Autodesk Fusion 360 part; units mm, degrees
(part 4 of 7)
extrude "USB nose reference rectangular stock" add sketch "USB nose reference rectangular stock sketch" along normal blind 1.1 separate body makes body 51 in component "USB A3 — GCT USB4720 shell drawing reconstruction"
fillet "USB nose reference corner rounds" radius 1.05 4 edges at (38.33, 1.55, 24.72) (46.67, 1.55, 24.72) (46.67, 1.55, 27.28) (38.33, 1.55, 27.28) on bodies 51 in component "USB A3 — GCT USB4720 shell drawing reconstruction"
combine "USB nose reference" operation add target body 50 tool bodies 51 in component "USB A3 — GCT USB4720 shell drawing reconstruction"
ref_plane "WorkPlane3" through (0, 2.1, 0) normal (0, 1, 0) x (0, 0, 1) in component "USB A3 — GCT USB4720 shell drawing reconstruction"
sketch "USB shell rear cavity simplified rectangular stock sketch" plane through (0, 2.1, 0) normal (0, 1, 0) x (1, 0, 0) in component "USB A3 — GCT USB4720 shell drawing reconstruction"
  line L0 (38.53, -27.43) -> (46.47, -27.43)
  line L1 (46.47, -27.43) -> (46.47, -24.57)
  line L2 (46.47, -24.57) -> (38.53, -24.57)
  line L3 (38.53, -24.57) -> (38.53, -27.43)
  dimension "d1272" = 38.53
  dimension "d1273" = 27.43
  dimension "d1274" = 7.94
  dimension "d1275" = 2.86
  constraint horizontal L0
  constraint vertical L1
  constraint horizontal L2
  constraint vertical L3
  measures "d1272" horizontal distance of origin L0.start
  measures "d1273" vertical distance of origin L0.start
  measures "d1274" horizontal distance of L0.start L0.end
  measures "d1275" vertical distance of L0.end L1.end
extrude "USB shell rear cavity simplified rectangular stock" add sketch "USB shell rear cavity simplified rectangular stock sketch" along normal blind 5.5 separate body makes body 52 in component "USB A3 — GCT USB4720 shell drawing reconstruction"
fillet "USB shell rear cavity simplified corner rounds" radius 0.85 4 edges at (38.53, 4.85, 24.57) (46.47, 4.85, 24.57) (46.47, 4.85, 27.43) (38.53, 4.85, 27.43) on bodies 52 in component "USB A3 — GCT USB4720 shell drawing reconstruction"
combine "USB shell rear cavity simplified" operation cut target body 50 tool bodies 52 in component "USB A3 — GCT USB4720 shell drawing reconstruction"
ref_plane "WorkPlane4" through (0, 0.9, 0) normal (0, 1, 0) x (0, 0, 1) in component "USB A3 — GCT USB4720 shell drawing reconstruction"
sketch "USB nose inner cavity simplified rectangular stock sketch" plane through (0, 0.9, 0) normal (0, 1, 0) x (1, 0, 0) in component "USB A3 — GCT USB4720 shell drawing reconstruction"
  line L0 (38.53, -27.08) -> (46.47, -27.08)
  line L1 (46.47, -27.08) -> (46.47, -24.92)
  line L2 (46.47, -24.92) -> (38.53, -24.92)
  line L3 (38.53, -24.92) -> (38.53, -27.08)
  dimension "d1282" = 38.53
  dimension "d1283" = 27.08
  dimension "d1284" = 7.94
  dimension "d1285" = 2.16
  constraint horizontal L0
  constraint vertical L1
  constraint horizontal L2
  constraint vertical L3
  measures "d1282" horizontal distance of origin L0.start
  measures "d1283" vertical distance of origin L0.start
  measures "d1284" horizontal distance of L0.start L0.end
  measures "d1285" vertical distance of L0.end L1.end
extrude "USB nose inner cavity simplified rectangular stock" add sketch "USB nose inner cavity simplified rectangular stock sketch" along normal blind 1.3 separate body makes body 53 in component "USB A3 — GCT USB4720 shell drawing reconstruction"
fillet "USB nose inner cavity simplified corner rounds" radius 0.85 4 edges at (38.53, 1.55, 24.92) (46.47, 1.55, 24.92) (46.47, 1.55, 27.08) (38.53, 1.55, 27.08) on bodies 53 in component "USB A3 — GCT USB4720 shell drawing reconstruction"
combine "USB nose inner cavity simplified" operation cut target body 50 tool bodies 53 in component "USB A3 — GCT USB4720 shell drawing reconstruction"
ref_plane "WorkPlane5" through (0, 0, 26.3) normal (0, 0, 1) x (1, 0, 0) in component "USB A3 — GCT USB4720 shell drawing reconstruction"
sketch "USB grounding wing reference sketch" plane through (0, 0, 26.3) normal (0, 0, 1) x (1, 0, 0) in component "USB A3 — GCT USB4720 shell drawing reconstruction"
  line L0 (36.85, 3.9) -> (38.38, 3.9)
  line L1 (38.38, 3.9) -> (38.38, 5.2)
  line L2 (38.38, 5.2) -> (36.85, 5.2)
  line L3 (36.85, 5.2) -> (36.85, 3.9)
  dimension "d1292" = 36.85
  dimension "d1293" = 3.9
  dimension "d1294" = 1.53
  dimension "d1295" = 1.3
  constraint horizontal L0
  constraint vertical L1
  constraint horizontal L2
  constraint vertical L3
  measures "d1292" horizontal distance of origin L0.start
  measures "d1293" vertical distance of origin L0.start
  measures "d1294" horizontal distance of L0.start L0.end
  measures "d1295" vertical distance of L0.end L1.end
extrude "USB grounding wing reference" add sketch "USB grounding wing reference sketch" along normal blind 0.3 bodies 50 in component "USB A3 — GCT USB4720 shell drawing reconstruction"
ref_plane "WorkPlane6" through (0, 0, 26.3) normal (0, 0, 1) x (1, 0, 0) in component "USB A3 — GCT USB4720 shell drawing reconstruction"
sketch "USB grounding wing reference sketch (1)" plane through (0, 0, 26.3) normal (0, 0, 1) x (1, 0, 0) in component "USB A3 — GCT USB4720 shell drawing reconstruction"
  line L0 (46.62, 3.9) -> (48.15, 3.9)
  line L1 (48.15, 3.9) -> (48.15, 5.2)
  line L2 (48.15, 5.2) -> (46.62, 5.2)
  line L3 (46.62, 5.2) -> (46.62, 3.9)
  dimension "d1300" = 46.62
  dimension "d1301" = 3.9
  dimension "d1302" = 1.53
  dimension "d1303" = 1.3
  constraint horizontal L0
  constraint vertical L1
  constraint horizontal L2
  constraint vertical L3
  measures "d1300" horizontal distance of origin L0.start
  measures "d1301" vertical distance of origin L0.start
  measures "d1302" horizontal distance of L0.start L0.end
  measures "d1303" vertical distance of L0.end L1.end
extrude "USB grounding wing reference (1)" add sketch "USB grounding wing reference sketch (1)" along normal blind 0.3 bodies 50 in component "USB A3 — GCT USB4720 shell drawing reconstruction"
ref_plane "WorkPlane7" through (0, 0, 26.3) normal (0, 0, 1) x (1, 0, 0) in component "USB A3 — GCT USB4720 shell drawing reconstruction"
sketch "USB grounding wing reference sketch (2)" plane through (0, 0, 26.3) normal (0, 0, 1) x (1, 0, 0) in component "USB A3 — GCT USB4720 shell drawing reconstruction"
  line L0 (36.85, 5.9) -> (38.38, 5.9)
  line L1 (38.38, 5.9) -> (38.38, 7.2)
  line L2 (38.38, 7.2) -> (36.85, 7.2)
  line L3 (36.85, 7.2) -> (36.85, 5.9)
  dimension "d1308" = 36.85
  dimension "d1309" = 5.9
  dimension "d1310" = 1.53
  dimension "d1311" = 1.3
  constraint horizontal L0
  constraint vertical L1
  constraint horizontal L2
  constraint vertical L3
  measures "d1308" horizontal distance of origin L0.start
  measures "d1309" vertical distance of origin L0.start
  measures "d1310" horizontal distance of L0.start L0.end
  measures "d1311" vertical distance of L0.end L1.end
extrude "USB grounding wing reference (2)" add sketch "USB grounding wing reference sketch (2)" along normal blind 0.3 bodies 50 in component "USB A3 — GCT USB4720 shell drawing reconstruction"
ref_plane "WorkPlane8" through (0, 0, 26.3) normal (0, 0, 1) x (1, 0, 0) in component "USB A3 — GCT USB4720 shell drawing reconstruction"
sketch "USB grounding wing reference sketch (3)" plane through (0, 0, 26.3) normal (0, 0, 1) x (1, 0, 0) in component "USB A3 — GCT USB4720 shell drawing reconstruction"
  line L0 (46.62, 5.9) -> (48.15, 5.9)
  line L1 (48.15, 5.9) -> (48.15, 7.2)
  line L2 (48.15, 7.2) -> (46.62, 7.2)
  line L3 (46.62, 7.2) -> (46.62, 5.9)
  dimension "d1316" = 46.62
  dimension "d1317" = 5.9
  dimension "d1318" = 1.53
  dimension "d1319" = 1.3
  constraint horizontal L0
  constraint vertical L1
  constraint horizontal L2
  constraint vertical L3
  measures "d1316" horizontal distance of origin L0.start
  measures "d1317" vertical distance of origin L0.start
  measures "d1318" horizontal distance of L0.start L0.end
  measures "d1319" vertical distance of L0.end L1.end
extrude "USB grounding wing reference (3)" add sketch "USB grounding wing reference sketch (3)" along normal blind 0.3 bodies 50 in component "USB A3 — GCT USB4720 shell drawing reconstruction"
ref_plane "WorkPlane1" through (0, 6.6, 0) normal (0, 1, 0) x (0, 0, 1) in component "USB A3 — tongue and rear insulator reference"
sketch "USB rear insulator rectangular stock sketch" plane through (0, 6.6, 0) normal (0, 1, 0) x (1, 0, 0) in component "USB A3 — tongue and rear insulator reference"
  line L0 (38.6, -27.05) -> (46.4, -27.05)
  line L1 (46.4, -27.05) -> (46.4, -24.95)
  line L2 (46.4, -24.95) -> (38.6, -24.95)
  line L3 (38.6, -24.95) -> (38.6, -27.05)
  dimension "d1324" = 38.6
  dimension "d1325" = 27.05
  dimension "d1326" = 7.8
  dimension "d1327" = 2.1
  constraint horizontal L0
  constraint vertical L1
  constraint horizontal L2
  constraint vertical L3
  measures "d1324" horizontal distance of origin L0.start
  measures "d1325" vertical distance of origin L0.start
  measures "d1326" horizontal distance of L0.start L0.end
  measures "d1327" vertical distance of L0.end L1.end
extrude "USB rear insulator rectangular stock" add sketch "USB rear insulator rectangular stock sketch" along normal blind 1 separate body makes body 54 in component "USB A3 — tongue and rear insulator reference"
fillet "USB rear insulator corner rounds" radius 0.5 4 edges at (38.6, 7.1, 24.95) (46.4, 7.1, 24.95) (46.4, 7.1, 27.05) (38.6, 7.1, 27.05) on bodies 54 in component "USB A3 — tongue and rear insulator reference"
ref_plane "WorkPlane2" through (0, 0, 25.65) normal (0, 0, 1) x (1, 0, 0) in component "USB A3 — tongue and rear insulator reference"
sketch "USB tongue6.69x0.70 reference sketch" plane through (0, 0, 25.65) normal (0, 0, 1) x (1, 0, 0) in component "USB A3 — tongue and rear insulator reference"
  line L0 (39.155, 1.2) -> (45.845, 1.2)
  line L1 (45.845, 1.2) -> (45.845, 6.6)
  line L2 (45.845, 6.6) -> (39.155, 6.6)
  line L3 (39.155, 6.6) -> (39.155, 1.2)
  dimension "d1334" = 39.155
  dimension "d1335" = 1.2
  dimension "d1336" = 6.69
  dimension "d1337" = 5.4
  constraint horizontal L0
  constraint vertical L1
  constraint horizontal L2
  constraint vertical L3
  measures "d1334" horizontal distance of origin L0.start
  measures "d1335" vertical distance of origin L0.start
  measures "d1336" horizontal distance of L0.start L0.end
  measures "d1337" vertical distance of L0.end L1.end
extrude "USB tongue6.69x0.70 reference" add sketch "USB tongue6.69x0.70 reference sketch" along normal blind 0.7 bodies 54 in component "USB A3 — tongue and rear insulator reference"
ref_plane "WorkPlane1" through (0, 1.2, 0) normal (0, 1, 0) x (0, 0, 1) in component "USB A3 — GCT LIM gasket nominal reference"
sketch "USB LIM gasket reference rectangular stock sketch" plane through (0, 1.2, 0) normal (0, 1, 0) x (1, 0, 0) in component "USB A3 — GCT LIM gasket nominal reference"
  line L0 (37.75, -27.86) -> (47.25, -27.86)
  line L1 (47.25, -27.86) -> (47.25, -24.14)
  line L2 (47.25, -24.14) -> (37.75, -24.14)
  line L3 (37.75, -24.14) -> (37.75, -27.86)
  dimension "d1342" = 37.75
  dimension "d1343" = 27.86
  dimension "d1344" = 9.5
  dimension "d1345" = 3.72
  constraint horizontal L0
  constraint vertical L1
  constraint horizontal L2
  constraint vertical L3
  measures "d1342" horizontal distance of origin L0.start
  measures "d1343" vertical distance of origin L0.start
  measures "d1344" horizontal distance of L0.start L0.end
  measures "d1345" vertical distance of L0.end L1.end
extrude "USB LIM gasket reference rectangular stock" add sketch "USB LIM gasket reference rectangular stock sketch" along normal blind 0.4 separate body makes body 55 in component "USB A3 — GCT LIM gasket nominal reference"
fillet "USB LIM gasket reference corner rounds" radius 1.5 4 edges at (37.75, 1.4, 24.14) (47.25, 1.4, 24.14) (47.25, 1.4, 27.86) (37.75, 1.4, 27.86) on bodies 55 in component "USB A3 — GCT LIM gasket nominal reference"
ref_plane "WorkPlane2" through (0, 1.19, 0) normal (0, 1, 0) x (0, 0, 1) in component "USB A3 — GCT LIM gasket nominal reference"
sketch "USB gasket inner shell clearance rectangular stock sketch" plane through (0, 1.19, 0) normal (0, 1, 0) x (1, 0, 0) in component "USB A3 — GCT LIM gasket nominal reference"
  line L0 (38.31, -27.3) -> (46.69, -27.3)
  line L1 (46.69, -27.3) -> (46.69, -24.7)
  line L2 (46.69, -24.7) -> (38.31, -24.7)
  line L3 (38.31, -24.7) -> (38.31, -27.3)
  dimension "d1352" = 38.31
  dimension "d1353" = 27.3
  dimension "d1354" = 8.38
  dimension "d1355" = 2.6
  constraint horizontal L0
  constraint vertical L1
  constraint horizontal L2
  constraint vertical L3
  measures "d1352" horizontal distance of origin L0.start
  measures "d1353" vertical distance of origin L0.start
  measures "d1354" horizontal distance of L0.start L0.end
  measures "d1355" vertical distance of L0.end L1.end
extrude "USB gasket inner shell clearance rectangular stock" add sketch "USB gasket inner shell clearance rectangular stock sketch" along normal blind 0.42 separate body makes body 56 in component "USB A3 — GCT LIM gasket nominal reference"
fillet "USB gasket inner shell clearance corner rounds" radius 1.07 4 edges at (38.31, 1.4, 24.7) (46.69, 1.4, 24.7) (46.69, 1.4, 27.3) (38.31, 1.4, 27.3) on bodies 56 in component "USB A3 — GCT LIM gasket nominal reference"
combine "USB gasket inner shell clearance" operation cut target body 55 tool bodies 56 in component "USB A3 — GCT LIM gasket nominal reference"
ref_plane "WorkPlane1" through (0, 0, 25.62) normal (0, 0, 1) x (1, 0, 0) in component "USB A3 — illustrative contact stripes"
sketch "USB visual contact stripe sketch" plane through (0, 0, 25.62) normal (0, 0, 1) x (1, 0, 0) in component "USB A3 — illustrative contact stripes"
  line L0 (40.625, 1.3) -> (40.875, 1.3)
  line L1 (40.875, 1.3) -> (40.875, 4)
  line L2 (40.875, 4) -> (40.625, 4)
  line L3 (40.625, 4) -> (40.625, 1.3)
  dimension "d1362" = 40.625
  dimension "d1363" = 1.3
  dimension "d1364" = 0.25
  dimension "d1365" = 2.7
  constraint horizontal L0
  constraint vertical L1
  constraint horizontal L2
  constraint vertical L3
  measures "d1362" horizontal distance of origin L0.start
  measures "d1363" vertical distance of origin L0.start
  measures "d1364" horizontal distance of L0.start L0.end
  measures "d1365" vertical distance of L0.end L1.end
extrude "USB visual contact stripe" add sketch "USB visual contact stripe sketch" along normal blind 0.03 separate body makes body 57 in component "USB A3 — illustrative contact stripes"
ref_plane "WorkPlane2" through (0, 0, 25.62) normal (0, 0, 1) x (1, 0, 0) in component "USB A3 — illustrative contact stripes"
sketch "USB visual contact stripe sketch (1)" plane through (0, 0, 25.62) normal (0, 0, 1) x (1, 0, 0) in component "USB A3 — illustrative contact stripes"
  line L0 (41.125, 1.3) -> (41.375, 1.3)
  line L1 (41.375, 1.3) -> (41.375, 4)
  line L2 (41.375, 4) -> (41.125, 4)
  line L3 (41.125, 4) -> (41.125, 1.3)
  dimension "d1370" = 41.125
  dimension "d1371" = 1.3
  dimension "d1372" = 0.25
  dimension "d1373" = 2.7
  constraint horizontal L0
  constraint vertical L1
  constraint horizontal L2
  constraint vertical L3
  measures "d1370" horizontal distance of origin L0.start
  measures "d1371" vertical distance of origin L0.start
  measures "d1372" horizontal distance of L0.start L0.end
  measures "d1373" vertical distance of L0.end L1.end
extrude "USB visual contact stripe (1)" add sketch "USB visual contact stripe sketch (1)" along normal blind 0.03 separate body makes body 58 in component "USB A3 — illustrative contact stripes"
ref_plane "WorkPlane3" through (0, 0, 25.62) normal (0, 0, 1) x (1, 0, 0) in component "USB A3 — illustrative contact stripes"
sketch "USB visual contact stripe sketch (2)" plane through (0, 0, 25.62) normal (0, 0, 1) x (1, 0, 0) in component "USB A3 — illustrative contact stripes"
  line L0 (41.625, 1.3) -> (41.875, 1.3)
  line L1 (41.875, 1.3) -> (41.875, 4)
  line L2 (41.875, 4) -> (41.625, 4)
  line L3 (41.625, 4) -> (41.625, 1.3)
  dimension "d1378" = 41.625
  dimension "d1379" = 1.3
  dimension "d1380" = 0.25
  dimension "d1381" = 2.7
  constraint horizontal L0
  constraint vertical L1
  constraint horizontal L2
  constraint vertical L3
  measures "d1378" horizontal distance of origin L0.start
  measures "d1379" vertical distance of origin L0.start
  measures "d1380" horizontal distance of L0.start L0.end
  measures "d1381" vertical distance of L0.end L1.end
extrude "USB visual contact stripe (2)" add sketch "USB visual contact stripe sketch (2)" along normal blind 0.03 separate body makes body 59 in component "USB A3 — illustrative contact stripes"
ref_plane "WorkPlane4" through (0, 0, 25.62) normal (0, 0, 1) x (1, 0, 0) in component "USB A3 — illustrative contact stripes"
sketch "USB visual contact stripe sketch (3)" plane through (0, 0, 25.62) normal (0, 0, 1) x (1, 0, 0) in component "USB A3 — illustrative contact stripes"
  line L0 (42.125, 1.3) -> (42.375, 1.3)
  line L1 (42.375, 1.3) -> (42.375, 4)
  line L2 (42.375, 4) -> (42.125, 4)
  line L3 (42.125, 4) -> (42.125, 1.3)
  dimension "d1386" = 42.125
  dimension "d1387" = 1.3
  dimension "d1388" = 0.25
  dimension "d1389" = 2.7
  constraint horizontal L0
  constraint vertical L1
  constraint horizontal L2
  constraint vertical L3
  measures "d1386" horizontal distance of origin L0.start
  measures "d1387" vertical distance of origin L0.start
  measures "d1388" horizontal distance of L0.start L0.end
  measures "d1389" vertical distance of L0.end L1.end
extrude "USB visual contact stripe (3)" add sketch "USB visual contact stripe sketch (3)" along normal blind 0.03 separate body makes body 60 in component "USB A3 — illustrative contact stripes"
ref_plane "WorkPlane5" through (0, 0, 25.62) normal (0, 0, 1) x (1, 0, 0) in component "USB A3 — illustrative contact stripes"
sketch "USB visual contact stripe sketch (4)" plane through (0, 0, 25.62) normal (0, 0, 1) x (1, 0, 0) in component "USB A3 — illustrative contact stripes"
  line L0 (42.625, 1.3) -> (42.875, 1.3)
  line L1 (42.875, 1.3) -> (42.875, 4)
  line L2 (42.875, 4) -> (42.625, 4)
  line L3 (42.625, 4) -> (42.625, 1.3)
  dimension "d1394" = 42.625
  dimension "d1395" = 1.3
  dimension "d1396" = 0.25
  dimension "d1397" = 2.7
  constraint horizontal L0
  constraint vertical L1
  constraint horizontal L2
  constraint vertical L3
  measures "d1394" horizontal distance of origin L0.start
  measures "d1395" vertical distance of origin L0.start
  measures "d1396" horizontal distance of L0.start L0.end
  measures "d1397" vertical distance of L0.end L1.end
extrude "USB visual contact stripe (4)" add sketch "USB visual contact stripe sketch (4)" along normal blind 0.03 separate body makes body 61 in component "USB A3 — illustrative contact stripes"
ref_plane "WorkPlane6" through (0, 0, 25.62) normal (0, 0, 1) x (1, 0, 0) in component "USB A3 — illustrative contact stripes"
sketch "USB visual contact stripe sketch (5)" plane through (0, 0, 25.62) normal (0, 0, 1) x (1, 0, 0) in component "USB A3 — illustrative contact stripes"
  line L0 (43.125, 1.3) -> (43.375, 1.3)
  line L1 (43.375, 1.3) -> (43.375, 4)
  line L2 (43.375, 4) -> (43.125, 4)
  line L3 (43.125, 4) -> (43.125, 1.3)
  dimension "d1402" = 43.125
  dimension "d1403" = 1.3
  dimension "d1404" = 0.25
  dimension "d1405" = 2.7
  constraint horizontal L0
  constraint vertical L1
  constraint horizontal L2
  constraint vertical L3
  measures "d1402" horizontal distance of origin L0.start
  measures "d1403" vertical distance of origin L0.start
  measures "d1404" horizontal distance of L0.start L0.end
  measures "d1405" vertical distance of L0.end L1.end
extrude "USB visual contact stripe (5)" add sketch "USB visual contact stripe sketch (5)" along normal blind 0.03 separate body makes body 62 in component "USB A3 — illustrative contact stripes"
ref_plane "WorkPlane7" through (0, 0, 25.62) normal (0, 0, 1) x (1, 0, 0) in component "USB A3 — illustrative contact stripes"
sketch "USB visual contact stripe sketch (6)" plane through (0, 0, 25.62) normal (0, 0, 1) x (1, 0, 0) in component "USB A3 — illustrative contact stripes"
  line L0 (43.625, 1.3) -> (43.875, 1.3)
  line L1 (43.875, 1.3) -> (43.875, 4)
  line L2 (43.875, 4) -> (43.625, 4)
  line L3 (43.625, 4) -> (43.625, 1.3)
  dimension "d1410" = 43.625
  dimension "d1411" = 1.3
  dimension "d1412" = 0.25
  dimension "d1413" = 2.7
  constraint horizontal L0
  constraint vertical L1
  constraint horizontal L2
  constraint vertical L3
  measures "d1410" horizontal distance of origin L0.start
  measures "d1411" vertical distance of origin L0.start
  measures "d1412" horizontal distance of L0.start L0.end
  measures "d1413" vertical distance of L0.end L1.end
extrude "USB visual contact stripe (6)" add sketch "USB visual contact stripe sketch (6)" along normal blind 0.03 separate body makes body 63 in component "USB A3 — illustrative contact stripes"
ref_plane "WorkPlane8" through (0, 0, 25.62) normal (0, 0, 1) x (1, 0, 0) in component "USB A3 — illustrative contact stripes"
sketch "USB visual contact stripe sketch (7)" plane through (0, 0, 25.62) normal (0, 0, 1) x (1, 0, 0) in component "USB A3 — illustrative contact stripes"
  line L0 (44.125, 1.3) -> (44.375, 1.3)
  line L1 (44.375, 1.3) -> (44.375, 4)
  line L2 (44.375, 4) -> (44.125, 4)
  line L3 (44.125, 4) -> (44.125, 1.3)
  dimension "d1418" = 44.125
  dimension "d1419" = 1.3
  dimension "d1420" = 0.25
  dimension "d1421" = 2.7
  constraint horizontal L0
  constraint vertical L1
  constraint horizontal L2
  constraint vertical L3
  measures "d1418" horizontal distance of origin L0.start
  measures "d1419" vertical distance of origin L0.start
  measures "d1420" horizontal distance of L0.start L0.end
  measures "d1421" vertical distance of L0.end L1.end
extrude "USB visual contact stripe (7)" add sketch "USB visual contact stripe sketch (7)" along normal blind 0.03 separate body makes body 64 in component "USB A3 — illustrative contact stripes"
ref_plane "WorkPlane9" through (0, 0, 26.35) normal (0, 0, 1) x (1, 0, 0) in component "USB A3 — illustrative contact stripes"
sketch "USB visual contact stripe sketch (8)" plane through (0, 0, 26.35) normal (0, 0, 1) x (1, 0, 0) in component "USB A3 — illustrative contact stripes"
  line L0 (40.625, 1.3) -> (40.875, 1.3)
  line L1 (40.875, 1.3) -> (40.875, 4)
  line L2 (40.875, 4) -> (40.625, 4)
  line L3 (40.625, 4) -> (40.625, 1.3)
  dimension "d1426" = 40.625
  dimension "d1427" = 1.3
  dimension "d1428" = 0.25
  dimension "d1429" = 2.7
  constraint horizontal L0
  constraint vertical L1
  constraint horizontal L2
  constraint vertical L3
  measures "d1426" horizontal distance of origin L0.start
  measures "d1427" vertical distance of origin L0.start
  measures "d1428" horizontal distance of L0.start L0.end
  measures "d1429" vertical distance of L0.end L1.end
extrude "USB visual contact stripe (8)" add sketch "USB visual contact stripe sketch (8)" along normal blind 0.03 separate body makes body 65 in component "USB A3 — illustrative contact stripes"
ref_plane "WorkPlane10" through (0, 0, 26.35) normal (0, 0, 1) x (1, 0, 0) in component "USB A3 — illustrative contact stripes"
sketch "USB visual contact stripe sketch (9)" plane through (0, 0, 26.35) normal (0, 0, 1) x (1, 0, 0) in component "USB A3 — illustrative contact stripes"
  line L0 (41.125, 1.3) -> (41.375, 1.3)
  line L1 (41.375, 1.3) -> (41.375, 4)
  line L2 (41.375, 4) -> (41.125, 4)
  line L3 (41.125, 4) -> (41.125, 1.3)
  dimension "d1434" = 41.125
  dimension "d1435" = 1.3
  dimension "d1436" = 0.25
  dimension "d1437" = 2.7
  constraint horizontal L0
  constraint vertical L1
  constraint horizontal L2
  constraint vertical L3
  measures "d1434" horizontal distance of origin L0.start
  measures "d1435" vertical distance of origin L0.start
  measures "d1436" horizontal distance of L0.start L0.end
  measures "d1437" vertical distance of L0.end L1.end
extrude "USB visual contact stripe (9)" add sketch "USB visual contact stripe sketch (9)" along normal blind 0.03 separate body makes body 66 in component "USB A3 — illustrative contact stripes"
ref_plane "WorkPlane11" through (0, 0, 26.35) normal (0, 0, 1) x (1, 0, 0) in component "USB A3 — illustrative contact stripes"
sketch "USB visual contact stripe sketch (10)" plane through (0, 0, 26.35) normal (0, 0, 1) x (1, 0, 0) in component "USB A3 — illustrative contact stripes"
  line L0 (41.625, 1.3) -> (41.875, 1.3)
  line L1 (41.875, 1.3) -> (41.875, 4)
  line L2 (41.875, 4) -> (41.625, 4)
  line L3 (41.625, 4) -> (41.625, 1.3)
  dimension "d1442" = 41.625
  dimension "d1443" = 1.3
  dimension "d1444" = 0.25
  dimension "d1445" = 2.7
  constraint horizontal L0
  constraint vertical L1
  constraint horizontal L2
  constraint vertical L3
  measures "d1442" horizontal distance of origin L0.start
  measures "d1443" vertical distance of origin L0.start
  measures "d1444" horizontal distance of L0.start L0.end
  measures "d1445" vertical distance of L0.end L1.end
extrude "USB visual contact stripe (10)" add sketch "USB visual contact stripe sketch (10)" along normal blind 0.03 separate body makes body 67 in component "USB A3 — illustrative contact stripes"
ref_plane "WorkPlane12" through (0, 0, 26.35) normal (0, 0, 1) x (1, 0, 0) in component "USB A3 — illustrative contact stripes"
sketch "USB visual contact stripe sketch (11)" plane through (0, 0, 26.35) normal (0, 0, 1) x (1, 0, 0) in component "USB A3 — illustrative contact stripes"
  line L0 (42.125, 1.3) -> (42.375, 1.3)
  line L1 (42.375, 1.3) -> (42.375, 4)
  line L2 (42.375, 4) -> (42.125, 4)
  line L3 (42.125, 4) -> (42.125, 1.3)
  dimension "d1450" = 42.125
  dimension "d1451" = 1.3
  dimension "d1452" = 0.25
  dimension "d1453" = 2.7
  constraint horizontal L0
  constraint vertical L1
  constraint horizontal L2
  constraint vertical L3
  measures "d1450" horizontal distance of origin L0.start
  measures "d1451" vertical distance of origin L0.start
  measures "d1452" horizontal distance of L0.start L0.end
  measures "d1453" vertical distance of L0.end L1.end
extrude "USB visual contact stripe (11)" add sketch "USB visual contact stripe sketch (11)" along normal blind 0.03 separate body makes body 68 in component "USB A3 — illustrative contact stripes"
ref_plane "WorkPlane13" through (0, 0, 26.35) normal (0, 0, 1) x (1, 0, 0) in component "USB A3 — illustrative contact stripes"
sketch "USB visual contact stripe sketch (12)" plane through (0, 0, 26.35) normal (0, 0, 1) x (1, 0, 0) in component "USB A3 — illustrative contact stripes"
  line L0 (42.625, 1.3) -> (42.875, 1.3)
  line L1 (42.875, 1.3) -> (42.875, 4)
  line L2 (42.875, 4) -> (42.625, 4)
  line L3 (42.625, 4) -> (42.625, 1.3)
  dimension "d1458" = 42.625
  dimension "d1459" = 1.3
  dimension "d1460" = 0.25
  dimension "d1461" = 2.7
  constraint horizontal L0
  constraint vertical L1
  constraint horizontal L2
  constraint vertical L3
  measures "d1458" horizontal distance of origin L0.start
  measures "d1459" vertical distance of origin L0.start
  measures "d1460" horizontal distance of L0.start L0.end
  measures "d1461" vertical distance of L0.end L1.end
extrude "USB visual contact stripe (12)" add sketch "USB visual contact stripe sketch (12)" along normal blind 0.03 separate body makes body 69 in component "USB A3 — illustrative contact stripes"
ref_plane "WorkPlane14" through (0, 0, 26.35) normal (0, 0, 1) x (1, 0, 0) in component "USB A3 — illustrative contact stripes"
sketch "USB visual contact stripe sketch (13)" plane through (0, 0, 26.35) normal (0, 0, 1) x (1, 0, 0) in component "USB A3 — illustrative contact stripes"
  line L0 (43.125, 1.3) -> (43.375, 1.3)
  line L1 (43.375, 1.3) -> (43.375, 4)
  line L2 (43.375, 4) -> (43.125, 4)
  line L3 (43.125, 4) -> (43.125, 1.3)
  dimension "d1466" = 43.125
  dimension "d1467" = 1.3
  dimension "d1468" = 0.25
  dimension "d1469" = 2.7
  constraint horizontal L0
  constraint vertical L1
  constraint horizontal L2
  constraint vertical L3
  measures "d1466" horizontal distance of origin L0.start
  measures "d1467" vertical distance of origin L0.start
  measures "d1468" horizontal distance of L0.start L0.end
  measures "d1469" vertical distance of L0.end L1.end
extrude "USB visual contact stripe (13)" add sketch "USB visual contact stripe sketch (13)" along normal blind 0.03 separate body makes body 70 in component "USB A3 — illustrative contact stripes"
ref_plane "WorkPlane15" through (0, 0, 26.35) normal (0, 0, 1) x (1, 0, 0) in component "USB A3 — illustrative contact stripes"
sketch "USB visual contact stripe sketch (14)" plane through (0, 0, 26.35) normal (0, 0, 1) x (1, 0, 0) in component "USB A3 — illustrative contact stripes"
  line L0 (43.625, 1.3) -> (43.875, 1.3)
  line L1 (43.875, 1.3) -> (43.875, 4)
  line L2 (43.875, 4) -> (43.625, 4)
  line L3 (43.625, 4) -> (43.625, 1.3)
  dimension "d1474" = 43.625
  dimension "d1475" = 1.3
  dimension "d1476" = 0.25
  dimension "d1477" = 2.7
  constraint horizontal L0
  constraint vertical L1
  constraint horizontal L2
  constraint vertical L3
  measures "d1474" horizontal distance of origin L0.start
  measures "d1475" vertical distance of origin L0.start
  measures "d1476" horizontal distance of L0.start L0.end
  measures "d1477" vertical distance of L0.end L1.end
extrude "USB visual contact stripe (14)" add sketch "USB visual contact stripe sketch (14)" along normal blind 0.03 separate body makes body 71 in component "USB A3 — illustrative contact stripes"
ref_plane "WorkPlane16" through (0, 0, 26.35) normal (0, 0, 1) x (1, 0, 0) in component "USB A3 — illustrative contact stripes"
sketch "USB visual contact stripe sketch (15)" plane through (0, 0, 26.35) normal (0, 0, 1) x (1, 0, 0) in component "USB A3 — illustrative contact stripes"
  line L0 (44.125, 1.3) -> (44.375, 1.3)
  line L1 (44.375, 1.3) -> (44.375, 4)
  line L2 (44.375, 4) -> (44.125, 4)
  line L3 (44.125, 4) -> (44.125, 1.3)
  dimension "d1482" = 44.125
  dimension "d1483" = 1.3
  dimension "d1484" = 0.25
  dimension "d1485" = 2.7
  constraint horizontal L0
  constraint vertical L1
  constraint horizontal L2
  constraint vertical L3
  measures "d1482" horizontal distance of origin L0.start
  measures "d1483" vertical distance of origin L0.start
  measures "d1484" horizontal distance of L0.start L0.end
  measures "d1485" vertical distance of L0.end L1.end
extrude "USB visual contact stripe (15)" add sketch "USB visual contact stripe sketch (15)" along normal blind 0.03 separate body makes body 72 in component "USB A3 — illustrative contact stripes"
ref_plane "WorkPlane44" through (0, -0.3, 0) normal (0, 1, 0) x (0, 0, 1) in component "01 Shape A housing"
sketch "Bottom tiny bezel aperture with0.2mm clearance rectangular stock sketch" plane through (0, -0.3, 0) normal (0, 1, 0) x (1, 0, 0) in component "01 Shape A housing"
  line L0 (35.3, -30.2) -> (49.7, -30.2)
  line L1 (49.7, -30.2) -> (49.7, -21.8)
  line L2 (49.7, -21.8) -> (35.3, -21.8)
  line L3 (35.3, -21.8) -> (35.3, -30.2)
  dimension "d1490" = 35.3
  dimension "d1491" = 30.2
  dimension "d1492" = 14.4
  dimension "d1493" = 8.4
  constraint horizontal L0
  constraint vertical L1
  constraint horizontal L2
  constraint vertical L3
  measures "d1490" horizontal distance of origin L0.start
  measures "d1491" vertical distance of origin L0.start
  measures "d1492" horizontal distance of L0.start L0.end
  measures "d1493" vertical distance of L0.end L1.end
extrude "Bottom tiny bezel aperture with0.2mm clearance rectangular stock" add sketch "Bottom tiny bezel aperture with0.2mm clearance rectangular stock sketch" along normal blind 2.8 separate body makes body 73 in component "01 Shape A housing"
fillet "Bottom tiny bezel aperture with0.2mm clearance corner rounds" radius 1 4 edges at (35.3, 1.1, 21.8) (49.7, 1.1, 21.8) (49.7, 1.1, 30.2) (35.3, 1.1, 30.2) on bodies 73 in component "01 Shape A housing"
combine "Bottom tiny bezel aperture with0.2mm clearance" operation cut target body 1 tool bodies 73 in component "01 Shape A housing"
ref_plane "WorkPlane45" through (0, 0, 17) normal (0, 0, 1) x (1, 0, 0) in component "01 Shape A housing"
sketch "Fixed USB cartridge support floor sketch" plane through (0, 0, 17) normal (0, 0, 1) x (1, 0, 0) in component "01 Shape A housing"
  line L0 (29.4, 2.3) -> (55.6, 2.3)
  line L1 (55.6, 2.3) -> (55.6, 22)
  line L2 (55.6, 22) -> (29.4, 22)
  line L3 (29.4, 22) -> (29.4, 2.3)
  dimension "d1500" = 29.4
  dimension "d1501" = 2.3
  dimension "d1502" = 26.2
  dimension "d1503" = 19.7
  constraint horizontal L0
  constraint vertical L1
  constraint horizontal L2
  constraint vertical L3
  measures "d1500" horizontal distance of origin L0.start
  measures "d1501" vertical distance of origin L0.start
  measures "d1502" horizontal distance of L0.start L0.end
  measures "d1503" vertical distance of L0.end L1.end
extrude "Fixed USB cartridge support floor" add sketch "Fixed USB cartridge support floor sketch" along normal blind 2 bodies 1 in component "01 Shape A housing"
ref_plane "WorkPlane20" through (0, 0, 31.2) normal (0, 0, 1) x (1, 0, 0) in component "02 Single rear cover"
sketch "USB inward retention key integral to rear cover sketch" plane through (0, 0, 31.2) normal (0, 0, 1) x (1, 0, 0) in component "02 Single rear cover"
  line L0 (37.4, 22.4) -> (47.6, 22.4)
  line L1 (47.6, 22.4) -> (47.6, 24.4)
  line L2 (47.6, 24.4) -> (37.4, 24.4)
  line L3 (37.4, 24.4) -> (37.4, 22.4)
  dimension "d1508" = 37.4
  dimension "d1509" = 22.4
  dimension "d1510" = 10.2
  dimension "d1511" = 2
  constraint horizontal L0
  constraint vertical L1
  constraint horizontal L2
  constraint vertical L3
  measures "d1508" horizontal distance of origin L0.start
  measures "d1509" vertical distance of origin L0.start
  measures "d1510" horizontal distance of L0.start L0.end
  measures "d1511" vertical distance of L0.end L1.end
extrude "USB inward retention key integral to rear cover" add sketch "USB inward retention key integral to rear cover sketch" along normal blind 9.7 bodies 4 in component "02 Single rear cover"
ref_plane "WorkPlane21" through (0, 0, 33.7) normal (0, 0, 1) x (1, 0, 0) in component "02 Single rear cover"
sketch "USB rearward retention pad integral to rear cover sketch" plane through (0, 0, 33.7) normal (0, 0, 1) x (1, 0, 0) in component "02 Single rear cover"
  line L0 (37.4, 20) -> (47.6, 20)
  line L1 (47.6, 20) -> (47.6, 24.4)
  line L2 (47.6, 24.4) -> (37.4, 24.4)
  line L3 (37.4, 24.4) -> (37.4, 20)
  dimension "d1516" = 37.4
  dimension "d1517" = 20
  dimension "d1518" = 10.2
  dimension "d1519" = 4.4
  constraint horizontal L0
  constraint vertical L1
  constraint horizontal L2
  constraint vertical L3
  measures "d1516" horizontal distance of origin L0.start
  measures "d1517" vertical distance of origin L0.start
  measures "d1518" horizontal distance of L0.start L0.end
  measures "d1519" vertical distance of L0.end L1.end
extrude "USB rearward retention pad integral to rear cover" add sketch "USB rearward retention pad integral to rear cover sketch" along normal blind 7.2 bodies 4 in component "02 Single rear cover"
ref_plane "WorkPlane1" through (0, 0, 3) normal (0, 0, 1) x (1, 0, 0) in component "Chamber / A3 top manifold with serial return"
sketch "Manifold outer CO pocket sketch" plane through (0, 0, 3) normal (0, 0, 1) x (1, 0, 0) in component "Chamber / A3 top manifold with serial return"
  line L0 (3, 130) -> (35, 130)
  line L1 (35, 130) -> (35, 167)
  line L2 (35, 167) -> (3, 167)
  line L3 (3, 167) -> (3, 130)
  dimension "d1524" = 3
  dimension "d1525" = 130
  dimension "d1526" = 32
  dimension "d1527" = 37
  constraint horizontal L0
  constraint vertical L1
  constraint horizontal L2
  constraint vertical L3
  measures "d1524" horizontal distance of origin L0.start
  measures "d1525" vertical distance of origin L0.start
  measures "d1526" horizontal distance of L0.start L0.end
  measures "d1527" vertical distance of L0.end L1.end
extrude "Manifold outer CO pocket" add sketch "Manifold outer CO pocket sketch" along normal blind 33 separate body makes body 74 in component "Chamber / A3 top manifold with serial return"
ref_plane "WorkPlane2" through (0, 0, 3) normal (0, 0, 1) x (1, 0, 0) in component "Chamber / A3 top manifold with serial return"
sketch "Manifold outer upper row sketch" plane through (0, 0, 3) normal (0, 0, 1) x (1, 0, 0) in component "Chamber / A3 top manifold with serial return"
  line L0 (13, 160.5) -> (72.5, 160.5)
  line L1 (72.5, 160.5) -> (72.5, 177)
  line L2 (72.5, 177) -> (13, 177)
  line L3 (13, 177) -> (13, 160.5)
  dimension "d1532" = 13
  dimension "d1533" = 160.5
  dimension "d1534" = 59.5
  dimension "d1535" = 16.5
  constraint horizontal L0
  constraint vertical L1
  constraint horizontal L2
  constraint vertical L3
  measures "d1532" horizontal distance of origin L0.start
  measures "d1533" vertical distance of origin L0.start
  measures "d1534" horizontal distance of L0.start L0.end
  measures "d1535" vertical distance of L0.end L1.end
extrude "Manifold outer upper row" add sketch "Manifold outer upper row sketch" along normal blind 33 bodies 74 in component "Chamber / A3 top manifold with serial return"
ref_plane "WorkPlane3" through (68, 0, 0) normal (1, 0, 0) x (0, 1, 0) in component "Chamber / A3 top manifold with serial return"
sketch "Upper sensor row inlet turn sketch" plane through (68, 0, 0) normal (1, 0, 0) x (0, 0, -1) in component "Chamber / A3 top manifold with serial return"
  circle A0 centre (-22, 165) radius 4.5
  dimension "d1541" = 165
  dimension "d1542" = 4.5
  measures "d1541" vertical distance of origin A0.centre
  measures "d1542" radius of A0
extrude "Upper sensor row inlet turn" add sketch "Upper sensor row inlet turn sketch" along normal blind 2.75 bodies 74 in component "Chamber / A3 top manifold with serial return"
ref_plane "WorkPlane4" through (0, 162.5, 0) normal (0, 1, 0) x (0, 0, 1) in component "Chamber / A3 top manifold with serial return"
sketch "Inlet rise outside dry AO2 connector sketch" plane through (0, 162.5, 0) normal (0, 1, 0) x (1, 0, 0) in component "Chamber / A3 top manifold with serial return"
  circle A0 centre (70.75, -22) radius 4.5
  dimension "d1547" = 70.75
  dimension "d1549" = 4.5
  measures "d1547" horizontal distance of origin A0.centre
  measures "d1549" radius of A0
extrude "Inlet rise outside dry AO2 connector" add sketch "Inlet rise outside dry AO2 connector sketch" along normal blind 2.5 bodies 74 in component "Chamber / A3 top manifold with serial return"
ref_plane "WorkPlane5" through (70.75, 0, 0) normal (1, 0, 0) x (0, 1, 0) in component "Chamber / A3 top manifold with serial return"
sketch "Viewer-left inlet duct sketch" plane through (70.75, 0, 0) normal (1, 0, 0) x (0, 0, -1) in component "Chamber / A3 top manifold with serial return"
  circle A0 centre (-22, 162.5) radius 4.5
  dimension "d1555" = 162.5
  dimension "d1556" = 4.5
  measures "d1555" vertical distance of origin A0.centre
  measures "d1556" radius of A0
extrude "Viewer-left inlet duct" add sketch "Viewer-left inlet duct sketch" along normal blind 11.25 bodies 74 in component "Chamber / A3 top manifold with serial return"
ref_plane "WorkPlane6" through (0, 0, 5) normal (0, 0, 1) x (1, 0, 0) in component "Chamber / A3 top manifold with serial return"
sketch "Wet CO pocket interior sketch" plane through (0, 0, 5) normal (0, 0, 1) x (1, 0, 0) in component "Chamber / A3 top manifold with serial return"
  line L0 (5, 132) -> (33, 132)
  line L1 (33, 132) -> (33, 165)
  line L2 (33, 165) -> (5, 165)
  line L3 (5, 165) -> (5, 132)
  dimension "d1561" = 5
  dimension "d1562" = 132
  dimension "d1563" = 28
  dimension "d1564" = 33
  constraint horizontal L0
  constraint vertical L1
  constraint horizontal L2
  constraint vertical L3
  measures "d1561" horizontal distance of origin L0.start
  measures "d1562" vertical distance of origin L0.start
  measures "d1563" horizontal distance of L0.start L0.end
  measures "d1564" vertical distance of L0.end L1.end
extrude "Wet CO pocket interior" cut sketch "Wet CO pocket interior sketch" along normal blind 43 bodies 74 in component "Chamber / A3 top manifold with serial return"
ref_plane "WorkPlane7" through (0, 0, 5) normal (0, 0, 1) x (1, 0, 0) in component "Chamber / A3 top manifold with serial return"
sketch "Wet humidity and MD62 row interior sketch" plane through (0, 0, 5) normal (0, 0, 1) x (1, 0, 0) in component "Chamber / A3 top manifold with serial return"
  line L0 (15, 162.5) -> (70.5, 162.5)
  line L1 (70.5, 162.5) -> (70.5, 175)
  line L2 (70.5, 175) -> (15, 175)
  line L3 (15, 175) -> (15, 162.5)
  dimension "d1569" = 15
  dimension "d1570" = 162.5
  dimension "d1571" = 55.5
  dimension "d1572" = 12.5
  constraint horizontal L0
  constraint vertical L1
  constraint horizontal L2
  constraint vertical L3
  measures "d1569" horizontal distance of origin L0.start
  measures "d1570" vertical distance of origin L0.start
  measures "d1571" horizontal distance of L0.start L0.end
  measures "d1572" vertical distance of L0.end L1.end
extrude "Wet humidity and MD62 row interior" cut sketch "Wet humidity and MD62 row interior sketch" along normal blind 43 bodies 74 in component "Chamber / A3 top manifold with serial return"
ref_plane "WorkPlane8" through (0, 0, 4.9) normal (0, 0, 1) x (1, 0, 0) in component "Chamber / A3 top manifold with serial return"
sketch "Full-depth inlet-to-outlet bypass barrier sketch" plane through (0, 0, 4.9) normal (0, 0, 1) x (1, 0, 0) in component "Chamber / A3 top manifold with serial return"
  line L0 (4.9, 158) -> (27.25, 158)
  line L1 (27.25, 158) -> (27.25, 162.6)
  line L2 (27.25, 162.6) -> (4.9, 162.6)
  line L3 (4.9, 162.6) -> (4.9, 158)
  dimension "d1577" = 4.9
  dimension "d1578" = 158
  dimension "d1579" = 22.35
  dimension "d1580" = 4.6
  constraint horizontal L0
  constraint vertical L1
  constraint horizontal L2
  constraint vertical L3
  measures "d1577" horizontal distance of origin L0.start
  measures "d1578" vertical distance of origin L0.start
  measures "d1579" horizontal distance of L0.start L0.end
  measures "d1580" vertical distance of L0.end L1.end
extrude "Full-depth inlet-to-outlet bypass barrier" add sketch "Full-depth inlet-to-outlet bypass barrier sketch" along normal blind 31.1 bodies 74 in component "Chamber / A3 top manifold with serial return"
ref_plane "WorkPlane9" through (0, 0, 4.9) normal (0, 0, 1) x (1, 0, 0) in component "Chamber / A3 top manifold with serial return"
sketch "Exhaust junction upper 2 mm wall extension sketch" plane through (0, 0, 4.9) normal (0, 0, 1) x (1, 0, 0) in component "Chamber / A3 top manifold with serial return"
  line L0 (4.9, 162.5) -> (12.1, 162.5)
  line L1 (12.1, 162.5) -> (12.1, 167)
  line L2 (12.1, 167) -> (4.9, 167)
  line L3 (4.9, 167) -> (4.9, 162.5)
  dimension "d1585" = 4.9
  dimension "d1586" = 162.5
  dimension "d1587" = 7.2
  dimension "d1588" = 4.5
  constraint horizontal L0
  constraint vertical L1
  constraint horizontal L2
  constraint vertical L3
  measures "d1585" horizontal distance of origin L0.start
  measures "d1586" vertical distance of origin L0.start
  measures "d1587" horizontal distance of L0.start L0.end
  measures "d1588" vertical distance of L0.end L1.end
extrude "Exhaust junction upper 2 mm wall extension" add sketch "Exhaust junction upper 2 mm wall extension sketch" along normal blind 31.1 bodies 74 in component "Chamber / A3 top manifold with serial return"
ref_plane "WorkPlane10" through (0, 0, 29) normal (0, 0, 1) x (1, 0, 0) in component "Chamber / A3 top manifold with serial return"
sketch "Rear return isolation above sensing-face sweep sketch" plane through (0, 0, 29) normal (0, 0, 1) x (1, 0, 0) in component "Chamber / A3 top manifold with serial return"
  line L0 (4.9, 149) -> (27.25, 149)
  line L1 (27.25, 149) -> (27.25, 158.1)
  line L2 (27.25, 158.1) -> (4.9, 158.1)
  line L3 (4.9, 158.1) -> (4.9, 149)
  dimension "d1593" = 4.9
  dimension "d1594" = 149
  dimension "d1595" = 22.35
  dimension "d1596" = 9.1
  constraint horizontal L0
  constraint vertical L1
  constraint horizontal L2
  constraint vertical L3
  measures "d1593" horizontal distance of origin L0.start
  measures "d1594" vertical distance of origin L0.start
  measures "d1595" horizontal distance of L0.start L0.end
  measures "d1596" vertical distance of L0.end L1.end
extrude "Rear return isolation above sensing-face sweep" add sketch "Rear return isolation above sensing-face sweep sketch" along normal blind 7 bodies 74 in component "Chamber / A3 top manifold with serial return"
ref_plane "WorkPlane11" through (0, 0, 28) normal (0, 0, 1) x (1, 0, 0) in component "Chamber / A3 top manifold with serial return"
sketch "Humidity compartment rear bypass baffle sketch" plane through (0, 0, 28) normal (0, 0, 1) x (1, 0, 0) in component "Chamber / A3 top manifold with serial return"
  line L0 (48, 162.4) -> (50, 162.4)
  line L1 (50, 162.4) -> (50, 175.1)
  line L2 (50, 175.1) -> (48, 175.1)
  line L3 (48, 175.1) -> (48, 162.4)
  dimension "d1601" = 48
  dimension "d1602" = 162.4
  dimension "d1603" = 2
  dimension "d1604" = 12.7
  constraint horizontal L0
  constraint vertical L1
  constraint horizontal L2
  constraint vertical L3
  measures "d1601" horizontal distance of origin L0.start
  measures "d1602" vertical distance of origin L0.start
  measures "d1603" horizontal distance of L0.start L0.end
  measures "d1604" vertical distance of L0.end L1.end
extrude "Humidity compartment rear bypass baffle" add sketch "Humidity compartment rear bypass baffle sketch" along normal blind 8 bodies 74 in component "Chamber / A3 top manifold with serial return"
ref_plane "WorkPlane12" through (70.65, 0, 0) normal (1, 0, 0) x (0, 1, 0) in component "Chamber / A3 top manifold with serial return"
sketch "Inlet bore sketch" plane through (70.65, 0, 0) normal (1, 0, 0) x (0, 0, -1) in component "Chamber / A3 top manifold with serial return"
  circle A0 centre (-22, 162.5) radius 2.5
  dimension "d1610" = 162.5
  dimension "d1611" = 2.5
  measures "d1610" vertical distance of origin A0.centre
  measures "d1611" radius of A0
extrude "Inlet bore" cut sketch "Inlet bore sketch" along normal blind 11.45 bodies 74 in component "Chamber / A3 top manifold with serial return"
ref_plane "WorkPlane13" through (0, 162.4, 0) normal (0, 1, 0) x (0, 0, 1) in component "Chamber / A3 top manifold with serial return"
sketch "Inlet rise bore sketch" plane through (0, 162.4, 0) normal (0, 1, 0) x (1, 0, 0) in component "Chamber / A3 top manifold with serial return"
  circle A0 centre (70.75, -22) radius 2.5
  dimension "d1616" = 70.75
  dimension "d1618" = 2.5
  measures "d1616" horizontal distance of origin A0.centre
  measures "d1618" radius of A0
extrude "Inlet rise bore" cut sketch "Inlet rise bore sketch" along normal blind 2.7 bodies 74 in component "Chamber / A3 top manifold with serial return"
ref_plane "WorkPlane14" through (67.9, 0, 0) normal (1, 0, 0) x (0, 1, 0) in component "Chamber / A3 top manifold with serial return"
sketch "Upper inlet turn bore sketch" plane through (67.9, 0, 0) normal (1, 0, 0) x (0, 0, -1) in component "Chamber / A3 top manifold with serial return"
  circle A0 centre (-22, 165) radius 2.5
  dimension "d1624" = 165
  dimension "d1625" = 2.5
  measures "d1624" vertical distance of origin A0.centre
  measures "d1625" radius of A0
extrude "Upper inlet turn bore" cut sketch "Upper inlet turn bore sketch" along normal blind 2.95 bodies 74 in component "Chamber / A3 top manifold with serial return"
ref_plane "WorkPlane15" through (2.9, 0, 0) normal (1, 0, 0) x (0, 1, 0) in component "Chamber / A3 top manifold with serial return"
sketch "Exhaust wall and return junction bore sketch" plane through (2.9, 0, 0) normal (1, 0, 0) x (0, 0, -1) in component "Chamber / A3 top manifold with serial return"
  circle A0 centre (-22, 162.5) radius 2.5
  dimension "d1631" = 162.5
  dimension "d1632" = 2.5
  measures "d1631" vertical distance of origin A0.centre
  measures "d1632" radius of A0
extrude "Exhaust wall and return junction bore" cut sketch "Exhaust wall and return junction bore sketch" along normal blind 4.7 bodies 74 in component "Chamber / A3 top manifold with serial return"
ref_plane "WorkPlane16" through (0, 0, 21.9) normal (0, 0, 1) x (1, 0, 0) in component "Chamber / A3 top manifold with serial return"
sketch "Exhaust return depth bore sketch" plane through (0, 0, 21.9) normal (0, 0, 1) x (1, 0, 0) in component "Chamber / A3 top manifold with serial return"
  circle A0 centre (7.5, 162.5) radius 2.5
  dimension "d1637" = 7.5
  dimension "d1638" = 162.5
  dimension "d1639" = 2.5
  measures "d1637" horizontal distance of origin A0.centre
  measures "d1638" vertical distance of origin A0.centre
  measures "d1639" radius of A0
extrude "Exhaust return depth bore" cut sketch "Exhaust return depth bore sketch" along normal blind 11.7 bodies 74 in component "Chamber / A3 top manifold with serial return"
ref_plane "WorkPlane17" through (0, 145.4, 0) normal (0, 1, 0) x (0, 0, 1) in component "Chamber / A3 top manifold with serial return"
sketch "Exhaust return from below face-sweep barrier sketch" plane through (0, 145.4, 0) normal (0, 1, 0) x (1, 0, 0) in component "Chamber / A3 top manifold with serial return"
  circle A0 centre (7.5, -33.5) radius 2.5
  dimension "d1644" = 7.5
  dimension "d1645" = 33.5
  dimension "d1646" = 2.5
  measures "d1644" horizontal distance of origin A0.centre
  measures "d1645" vertical distance of origin A0.centre
  measures "d1646" radius of A0